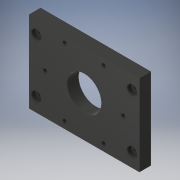
# Autodesk Inventor part: GA08
Saved by Autodesk Inventor 2017 (Build 210142000, 142)
## iProperties
Created: 2018-11-17
Part Number: GA08
Material: ABS Plastic
Document SubType Name: Modeling
Designer: Dell
Density: 1.06 g/cm^3
Appearance: Smooth - Black
Author: Dell
Autodesk Inventor part; units mm, degrees
ref_plane "YZ Plane" through (0, 0, 0) normal (1, 0, 0) x (0, 1, 0)
ref_plane "XZ Plane" through (0, 0, 0) normal (0, 1, 0) x (-1, 0, 0)
ref_plane "XY Plane" through (0, 0, 0) normal (0, 0, 1) x (1, 0, 0)
sketch "Sketch1" plane through (0, 0, 0) normal (0, 0, 1) x (1, 0, 0)
  line L0 (0, 0) -> (144, 0)
  line L1 (144, 0) -> (144, 106)
  line L2 (144, 106) -> (0, 106)
  line L3 (0, 106) -> (0, 0)
  line L4 (21, 53) -> (46.5, 97.1673) construction
  line L5 (46.5, 97.1673) -> (97.5, 97.1673) construction
  line L6 (97.5, 97.1673) -> (123, 53) construction
  line L7 (123, 53) -> (97.5, 8.8327) construction
  line L8 (97.5, 8.8327) -> (46.5, 8.8327) construction
  line L9 (46.5, 8.8327) -> (21, 53) construction
  circle A0 centre (21, 53) radius 2.5
  circle A1 centre (46.5, 8.8327) radius 2.5
  circle A2 centre (97.5, 8.8327) radius 2.5
  circle A3 centre (123, 53) radius 2.5
  circle A4 centre (97.5, 97.1673) radius 2.5
  circle A5 centre (46.5, 97.1673) radius 2.5
  line L10 (9.5, 88) -> (9.5, 18) construction
  circle A6 centre (9.5, 88) radius 2.5
  circle A7 centre (9.5, 18) radius 2.5
  line L11 (134.5, 88) -> (134.5, 18) construction
  circle A8 centre (134.5, 88) radius 2.5
  circle A9 centre (134.5, 18) radius 2.5
  circle A10 centre (72, 53) radius 22.5
  point P0 (72, 106)
  point P1 (144, 53)
  point P2 (9.5, 53)
  point P3 (134.5, 53)
  dimension "d0" = 144
  dimension "d1" = 106
  dimension "d2" = 5
  dimension "d3" = 51
  dimension "d6" = 360
  dimension "d8" = 70
  dimension "d9" = 9.5
  dimension "d10" = 5
  dimension "d11" = 5
  dimension "d12" = 9.5
  dimension "d13" = 5
  dimension "d14" = 5
  dimension "d15" = 45
  constraints: 24 end point, 11 centre point, 6 coincident, 5 horizontal alignment, 4 midpoint, 2 parallel, 2 vertical, 1 horizontal, 1 perpendicular, 1 vertical alignment, 26 other
  measures "d0" distance of L2.end L1.end
  measures "d1" distance of L1.end L0.end
  measures "d2" diameter of A0
  measures "d3" distance of L4.start point (72, 53)
  measures "d8" distance of L10.start L10.end
  measures "d9" distance between parallel lines of L3 L10
  measures "d10" diameter of A6
  measures "d11" diameter of A7
  measures "d12" distance between parallel lines of L1 L11
  measures "d13" diameter of A8
  measures "d14" diameter of A9
  measures "d15" diameter of A10
extrude "Extrusion1" add sketch "Sketch1" along normal blind 15
sketch "Sketch2" plane through (0, 0, 15) normal (0, 0, 1) x (1, 0, 0)
  circle A0 centre (46.5, 97.1673) radius 2.5 construction
  circle A1 centre (46.5, 97.1673) radius 6.5
  circle A2 centre (72, 53) radius 22.5 construction
  circle A3 centre (9.5, 88) radius 2.5 construction
  circle A4 centre (9.5, 18) radius 2.5 construction
  circle A5 centre (134.5, 88) radius 2.5 construction
  circle A6 centre (134.5, 18) radius 2.5 construction
  circle A7 centre (9.5, 88) radius 6.5
  circle A8 centre (9.5, 18) radius 6.5
  circle A9 centre (134.5, 18) radius 6.5
  circle A10 centre (134.5, 88) radius 6.5
  circle A11 centre (21, 53) radius 6.5
  circle A12 centre (46.5, 8.8327) radius 6.5
  circle A13 centre (97.5, 8.8327) radius 6.5
  circle A14 centre (123, 53) radius 6.5
  circle A15 centre (97.5, 97.1673) radius 6.5
  point P0 (0, 0)
  dimension "d18" = 13
  dimension "d19" = 13
  dimension "d20" = 13
  dimension "d21" = 13
  dimension "d22" = 13
  dimension "d25" = 360
  constraints: 10 centre point, 5 coincident, 13 other
  measures "d18" diameter of A1
  measures "d19" diameter of A7
  measures "d20" diameter of A8
  measures "d21" diameter of A9
  measures "d22" diameter of A10
extrude "Extrusion2" cut sketch "Sketch2" against normal blind 5 contours A7 | A8 | A9 | A10
body "Solid1"
